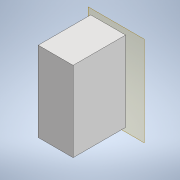
# Autodesk Inventor part: Display_Cover
Saved by Autodesk Inventor 2021 (Build 250183000, 183)
## iProperties
Created: 2020-08-10
Part Number: Display_Cover
Material: Generic
Document SubType Name: Modeling
Designer: ridvansong
Density: 1 g/cm^3
Appearance: Default
Author: ridvansong
Autodesk Inventor part; units mm, degrees
ref_plane "YZ Plane" through (0, 0, 0) normal (1, 0, 0) x (0, 1, 0)
ref_plane "XZ Plane" through (0, 0, 0) normal (0, 1, 0) x (-1, 0, 0)
ref_plane "XY Plane" through (0, 0, 0) normal (0, 0, 1) x (1, 0, 0)
ref_plane "Work Plane1" through (0, 0, 0) normal (0, 0, 1) x (1, 0, 0)
sketch "Sketch1" plane through (0, 0, 0) normal (0, 0, 1) x (1, 0, 0)
  line L0 (11.775, 18.625) -> (-4.025, 18.625) projected
  line L1 (11.775, 43.875) -> (11.775, 18.625) projected
  line L2 (-4.025, 43.875) -> (11.775, 43.875) projected
  line L3 (-4.025, 18.625) -> (-4.025, 43.875) projected
  line L4 (7.775, 43.875) -> (7.775, -42.625) projected
  line L5 (-4.025, 18.625) -> (6.775, 18.625)
  line L6 (6.775, 18.625) -> (6.775, 43.375)
  line L7 (6.775, 43.375) -> (-4.025, 43.375)
  line L8 (-4.025, 43.375) -> (-4.025, 18.625)
  circle A0 centre (1.775, 30.625) radius 1.1 projected
  point P0 (0, 0)
  point P1 (-4.025, 43.375)
  dimension "d0" = 0.5
  dimension "d1" = 1
  constraints: 8 end point, 2 collinear, 2 parallel, 1 horizontal, 1 perpendicular
  measures "d0" distance between parallel lines of L2 L7
  measures "d1" distance between parallel lines of L4 L6
ref_plane "Work Plane2" through (-11.525, -42.375, 16.25) normal (0, 0, 1) x (1, 0, 0)
extrude "Extrusion1" add sketch "Sketch1" along normal up to surface (16.25 mm away) contours L0 L3 L7 L6 | A0
sketch "Sketch2" plane through (-4.025, 43.375, 16.25) normal (0, 0, 1) x (1, 0, 0)
  line L0 (0, -85.75) -> (-7.5, -85.75)
  line L1 (-7.5, -85.75) -> (-7.5, 0)
  line L2 (-7.5, 0) -> (10.8, 0)
  line L3 (10.8, -24.75) -> (10.8, 0) projected
  line L4 (10.8, 0) -> (10.8, -24.75)
  line L5 (0, -24.75) -> (10.8, -24.75) projected
  line L6 (10.8, -24.75) -> (0, -24.75)
  line L7 (0, -24.75) -> (0, -64.5)
  line L8 (0, -64.5) -> (-1.85, -64.5)
  line L9 (-1.85, -64.5) -> (-1.85, -75.5)
  line L10 (-1.85, -75.5) -> (0, -75.5)
  line L11 (0, -75.5) -> (0, -85.75)
  line L12 (-7.5, -85.75) -> (6.5, -85.75) projected
  line L13 (-7.5, 0.25) -> (-7.5, -85.75) projected
  line L14 (0, -64.75) -> (0, -75.25) projected
  line L15 (0, -64.75) -> (-1.6, -64.75) projected
  line L16 (-1.6, -75.25) -> (-1.6, -64.75) projected
  line L17 (0, -75.25) -> (-1.6, -75.25) projected
  line L18 (0, -9.75) -> (0, -20.25) projected
  line L19 (0, -9.75) -> (-1.6, -9.75) projected
  line L20 (-1.6, -20.25) -> (-1.6, -9.75) projected
  line L21 (0, -20.25) -> (-1.6, -20.25) projected
  line L22 (-1.85, -9.5) -> (0.25, -9.5)
  line L23 (0.25, -9.5) -> (0.25, -20.5)
  line L24 (0.25, -20.5) -> (-1.85, -20.5)
  line L25 (-1.85, -20.5) -> (-1.85, -9.5)
  line L26 (0, 0) -> (10.8, 0) projected
  point P0 (4.025, -43.375)
  dimension "d4" = 0.25
  dimension "d5" = 0.25
  dimension "d6" = 0.25
  dimension "d7" = 0.25
  constraints: 28 end point, 7 perpendicular, 5 collinear, 1 horizontal, 1 point on line, 3 other
  measures "d4" distance between parallel lines of L20 L25
  measures "d5" distance between parallel lines of L9 L16
  measures "d6" distance between parallel lines of L15 L8
  measures "d7" distance between parallel lines of L17 L10
ref_plane "Work Plane3" through (-12.525, -42.875, 17.75) normal (0, 0, 1) x (1, 0, 0)
extrude "Extrusion2" add sketch "Sketch2" along normal up to surface (1.5 mm away) contours L0 L1 L2 L3 L5 L7 L8 L9 L10 L11
sketch "Sketch3" plane through (-11.525, 43.375, 17.75) normal (0, 0, 1) x (1, 0, 0)
  line L0 (18.3, 0) -> (18.3, -24.75) projected
  line L1 (18.3, -24.75) -> (7.5, -24.75) projected
  point P0 (11.525, -43.375)
  point P1 (13.3, -12.75)
  dimension "d13" = 5
  dimension "d14" = 12
  measures "d13" distance from line of L0 point (13.3, -12.75)
  measures "d14" distance from line of L1 point (13.3, -12.75)
hole "Hole1" at (1.775, 30.625, 17.75) direction (0, 0, -1) diameter 3.2 end through all counterbore diameter 6 counterbore depth 16.5
body "Solid1"
